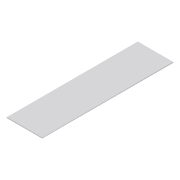
# Autodesk Inventor part: End Clear Ramp Surface 125 - Version 2
Saved by Autodesk Inventor 2015 (Build 190159000, 159)
## iProperties
Created: 2015-01-20
Part Number: End Clear Ramp Surface 125 - Version 2
Material: Generic
Document SubType Name: Modeling
Designer: Peter
Density: 1 g/cm^3
Appearance: Polycarbonate - Clear
Author: Peter
Autodesk Inventor part; units mm, degrees
ref_plane "YZ Plane" through (0, 0, 0) normal (1, 0, 0) x (0, 1, 0)
ref_plane "XZ Plane" through (0, 0, 0) normal (0, 1, 0) x (-1, 0, 0)
ref_plane "XY Plane" through (0, 0, 0) normal (0, 0, 1) x (1, 0, 0)
sketch "Sketch1" plane through (0, 0, 0) normal (0, 0, 1) x (1, 0, 0)
  line L0 (0, 0) -> (137.16, 0)
  line L1 (137.16, 0) -> (137.16, 3.175)
  line L2 (137.16, 3.175) -> (0, 3.175)
  line L3 (0, 3.175) -> (0, 0)
  dimension "d0" = 3.175
  dimension "d1" = 137.16
  constraints: 8 end point, 2 parallel, 1 horizontal, 1 perpendicular
  measures "d0" distance of L2.end L0.start
  measures "d1" distance of L1.end L2.end
extrude "Extrusion1" add sketch "Sketch1" along normal blind 508
body "Solid1"
